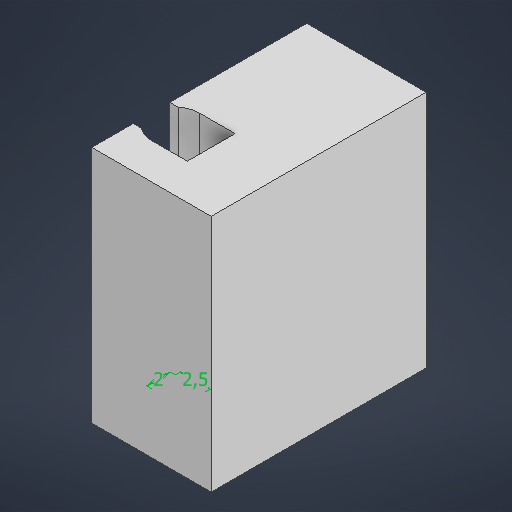
# Autodesk Inventor part: basebody
Saved by Autodesk Inventor 2026.1 (Build 301233020, 233B)
## iProperties
Created: 2025-12-12
Part Number: basebody
Material: Generic
Document SubType Name: Modeling
Designer: alexa
Density: 1 g/cm^3
Appearance: Default
Author: alexa
Autodesk Inventor part; units mm, degrees
ref_plane "YZ Plane" through (0, 0, 0) normal (1, 0, 0) x (0, 1, 0)
ref_plane "XZ Plane" through (0, 0, 0) normal (0, 1, 0) x (-1, 0, 0)
ref_plane "XY Plane" through (0, 0, 0) normal (0, 0, 1) x (1, 0, 0)
sketch "Sketch1" plane through (0, 0, 0) normal (0, 1, 0) x (-1, 0, 0)
  point P0 (0, 0)
sketch "Sketch2" plane through (0, 0, 0) normal (0, 1, 0) x (-1, 0, 0)
  line L0 (0, 0) -> (-5, 0)
  line L1 (-5, 0) -> (-5, -4)
  line L2 (-5, -4) -> (0, -4)
  line L3 (0, -4) -> (0, 0)
  line L4 (0, 0) -> (-10, 0)
  line L5 (-10, 0) -> (-10, -15)
  line L6 (-10, -15) -> (0, -15)
  line L7 (0, -15) -> (0, 0)
  circle A0 centre (-2, -2) radius 2
  point P0 (-2, 0)
  point P1 (0, -2)
  point P2 (-2, -4)
  dimension "d0" = 5
  dimension "d1" = 4
  dimension "d2" = 10
  dimension "d3" = 15
  constraints: 16 end point, 4 parallel, 3 tangent, 2 horizontal, 2 perpendicular, 1 centre point
  measures "d0" distance of L2.end L1.end
  measures "d1" distance of L1.end L0.end
  measures "d2" distance of L6.end L5.end
  measures "d3" distance of L5.end L4.end
sketch "Sketch3" plane through (0, 0, 0) normal (0, 1, 0) x (-1, 0, 0)
  line L0 (0, 0) -> (0, -4.0004)
  line L1 (0, -4.0004) -> (0, -2.0004)
  line L2 (0, -4.0004) -> (-2.5, -4.0004)
  dimension "d4" = 2
  dimension "d5" = 2.5
  constraints: 6 end point, 1 perpendicular, 1 point on line, 1 vertical
  measures "d4" distance of L0.end L1.end
  measures "d5" distance of L0.end L2.end
extrude "Extrusion1" add sketch "Sketch2" along normal blind 20 contours L3 A0 L0 | L3 L2 A0 | L1 L2 L7 L6 L5 L4
sketch "Sketch4" plane through (5, 0, 0) normal (0, 0, 1) x (1, 0, 0)
  line L0 (-5, 0) -> (-5, 20) projected
  line L1 (-5, 20) -> (5, 20)
  line L2 (5, 20) -> (5, 0)
  line L3 (5, 0) -> (-5, 0)
  line L4 (-5, 0) -> (-5, 20)
  constraints: 8 end point, 2 parallel, 1 horizontal, 1 perpendicular
extrude "Extrusion2" add sketch "Sketch4" along normal blind 3
sketch "Sketch5" plane through (0, 0, 0) normal (0, -1, 0) x (1, 0, 0)
  arc A0 (2, 0) -> (0, -2) centre (2, -2) ccw projected
  line L0 (0, -3.5296) -> (0, -0.4704)
  line L1 (0, -0.4704) -> (1.4533, -0.4704)
  line L2 (1.4533, -0.4704) -> (1.4533, -3.5296)
  line L3 (1.4533, -3.5296) -> (0, -3.5296)
  line L4 (0, -3.5296) -> (0, -0.4704)
  point P0 (0, 0)
  point P1 (0.7115, -0.4704)
  constraints: 10 end point, 2 parallel, 1 horizontal, 1 midpoint, 1 perpendicular, 1 tangent, 1 vertical
extrude "Extrusion3" cut sketch "Sketch5" against normal blind 200 contours L1 L2 L3 L0 A0
sketch "Sketch6" plane through (0, 0, 0) normal (0, -1, 0) x (1, 0, 0)
  line L0 (0, -2) -> (0, 3) projected
  line L1 (0, -0.4704) -> (1.2121, -0.4704)
  line L2 (1.2121, -0.4704) -> (1.2121, -2.1829)
  line L3 (1.2121, -2.1829) -> (0, -2.1829)
  line L4 (0, -2.1829) -> (0, -0.4704)
  point P0 (0, 0)
  constraints: 8 end point, 2 parallel, 1 horizontal, 1 perpendicular, 1 point on line
extrude "Extrusion4" cut sketch "Sketch6" against normal blind 200
body "Solid1"
